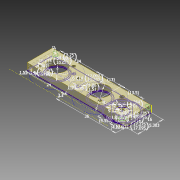
# Autodesk Inventor part: mount
Saved by Autodesk Inventor 2014 (Build 180170000, 170)
## iProperties
Created: 2013-09-13
Part Number: mount
Material: Nylon 6/6
Document SubType Name: Modeling
Designer: Brandon
Density: 1 g/cm^3
Appearance: Nylon 6
Author: Brandon
Autodesk Inventor part; units mm, degrees
ref_plane "YZ Plane" through (0, 0, 0) normal (1, 0, 0) x (0, 1, 0)
ref_plane "XZ Plane" through (0, 0, 0) normal (0, 1, 0) x (-1, 0, 0)
ref_plane "XY Plane" through (0, 0, 0) normal (0, 0, 1) x (1, 0, 0)
sketch "Sketch1" plane through (0, 0, 0) normal (0, 0, 1) x (1, 0, 0)
  circle A0 centre (0, 0) radius 0.88
  circle A1 centre (-13, 0) radius 6.031
  line L0 (0, 8.1062) -> (0, -7.1967)
  line L1 (-24, -7.1967) -> (0, -7.1967)
  line L2 (-24, 8.1062) -> (-24, -7.1967)
  circle A2 centre (-13, 0) radius 5.1925
  line L3 (-13, 0) -> (-9.1435, 0) construction
  line L4 (-13, 0) -> (-13, 0) construction
  circle A3 centre (-7.9046, 5.0954) radius 0.8375
  circle A4 centre (-18.0954, -5.0954) radius 0.8375
  circle A5 centre (13, 0) radius 6.031
  circle A6 centre (13, 0) radius 5.1925
  line L5 (13, 0) -> (9.1435, 0) construction
  line L6 (13, 0) -> (13, 0) construction
  circle A7 centre (7.9046, 5.0954) radius 0.8375
  circle A8 centre (18.0954, -5.0954) radius 0.8375
  line L7 (13, 0) -> (-13, 0)
  circle A9 centre (26.5, 0) radius 4.5 construction
  circle A10 centre (26.5, 0) radius 8.6375
  line L8 (26.5, 0) -> (30.5894, 0) construction
  circle A11 centre (22.8938, 3.6062) radius 1.132
  circle A12 centre (30.1062, -3.6062) radius 1.132
  line L9 (0, -7.1967) -> (-0.0026, -8.7967) construction
  line L10 (-0.0026, -8.7967) -> (-19.5634, -8.7649) construction
  line L11 (-0.0026, -8.7967) -> (19.5499, -8.8284) construction
  circle A13 centre (13, 0) radius 9 construction
  circle A14 centre (26.5, 0) radius 3.2675
  line L12 (13, 0) -> (26.5, 0)
  line L13 (30.1062, -3.6062) -> (22.8938, 3.6062) construction
  line L14 (33.2882, -0.4243) -> (26.0757, 6.7882)
  line L15 (19.7118, 0.4243) -> (26.9243, -6.7882)
  arc A15 (26.9243, -6.7882) -> (33.2882, -0.4243) centre (30.1062, -3.6062) ccw
  arc A16 (26.0757, 6.7882) -> (19.7118, 0.4243) centre (22.8938, 3.6062) ccw
  circle A17 centre (26.5, 0) radius 8
  circle A18 centre (26.5, 0) radius 3.5
  line L16 (-24, 8.1062) -> (0, 8.1062)
  line L17 (36, 8.1062) -> (36, -7.1967)
  line L18 (21.7235, -7.1967) -> (31.2765, -7.1967) construction
  line L19 (-0.0026, -8.7967) -> (-0.0018, -11.9967) construction
  line L20 (-0.0018, -11.9967) -> (30.0022, -11.9889) construction
  line L21 (-0.0018, -11.9967) -> (-29.9998, -12.0044) construction
  line L22 (-0.0018, -11.9967) -> (29.9963, -11.9967) construction
  circle A19 centre (0, 0) radius 4 construction
  line L23 (-13, 0) -> (-8.7354, 4.2646) construction
  line L24 (-13, 0) -> (-17.2646, -4.2646) construction
  line L25 (-8.7354, 4.2646) -> (-7.9046, 5.0954) construction
  line L26 (-17.2646, -4.2646) -> (-18.0954, -5.0954) construction
  line L27 (-17.2646, -4.2646) -> (-16.0896, -4.2646) construction
  circle A20 centre (13, 0) radius 12 construction
  circle A21 centre (-13, 0) radius 12 construction
  line L28 (1, 0) -> (-1, 0) construction
  line L29 (-19.031, 0) -> (-24, 0) construction
  line L30 (0, 8.1062) -> (36, 8.1062)
  line L31 (0, -7.1967) -> (36, -7.1967)
  line L32 (36, -7.1967) -> (36, -11.3938) construction
  circle A22 centre (22.8938, 3.6062) radius 1.9
  circle A23 centre (30.1062, -3.6062) radius 1.9
  dimension "d105" = 24
  dimension "d106" = 24
  dimension "d0" = 1.5
  dimension "d3" = 11.6
  dimension "d8" = 10
  dimension "d14" = 1.55
  dimension "d26" = 17
  dimension "d31" = 2
  dimension "d32" = 2
  dimension "d40" = 6.15
  dimension "d42" = 13
  dimension "d52" = 13.5
  dimension "d53" = 9
  dimension "d54" = 7
  dimension "d81" = 1.6
  dimension "d86" = 3.2
  dimension "d87" = 45
  dimension "d88" = 10.2
  dimension "d89" = 8
  dimension "d91" = 1.175
  dimension "d92" = 135
  dimension "d103" = 18
  dimension "d104" = 9
  dimension "d107" = 2
  dimension "d108" = 4.969
  dimension "d117" = 24
  dimension "d118" = 24
  dimension "d119" = 36
  dimension "d131" = 16
  dimension "d132" = 9.5529
  dimension "d133" = 4.7236
  dimension "d134" = 15.3029
  dimension "d135" = 3.8
  dimension "d136" = 3.8
  constraints: 68 end point, 22 centre point, 15 coincident, 10 horizontal, 9 point on circle, 7 collinear, 7 point on line, 7 tangent, 6 perpendicular, 6 symmetric about line, 3 equal length, 2 horizontal alignment, 2 midpoint, 1 equal radius, 1 parallel, 9 other
  measures "d42" distance of point (0, 0) A5.centre
  measures "d52" distance of L12.start L8.start
  measures "d53" diameter of A16
  measures "d54" diameter of A18
  measures "d81" distance of L9.end L0.end
  measures "d86" distance of L9.end L19.end
  measures "d87" angle of L8 L13
  measures "d88" distance of L13.start L13.end
  measures "d89" diameter of A19
  measures "d91" distance of L24.end L26.end
  measures "d92" angle of L26 L27
  measures "d103" diameter of A13
  measures "d104" diameter of A9
  measures "d107" distance of L28.start L28.end
  measures "d108" distance of L29.start L29.end
  measures "d117" distance of L2.start L0.start
  measures "d118" distance of L1.start L0.end
  measures "d119" distance of L0.end L17.end
  measures "d131" diameter of A17
  measures "d132" distance of L18.end L18.start
  measures "d133" distance of L17.end L18.end
  measures "d134" distance of L17.start L17.end
  measures "d135" diameter of A22
  measures "d136" diameter of A23
extrude "Extrusion5" add sketch "Sketch1" along normal blind 4 contours L7 L0 A0 | L7 A5 A10 L31 L0 A0 | A0 L0 L30 A16 A10 A5 L7 | A0 L0 L7 | L0 L7 A0 | A0 L0 L1 L2 L16 | A0 L7 L0 | L7 A6 A10 A5 | A5 A10 A6 L7 | A10 A16 A5 | A5 A17 L12 A6 A10 | A10 A6 L12 A17 A5 | A5 A17 L31 A10 | L30 A10 A16 | A16 A10 | A16 A17 A5 | A16 A10 A17 | A17 L12 A5 | A5 L12 L15 A15 L31 A17 | A10 L30 A15 A17 A16 | A17 A16 L15 L12 A5 | A5 L12 A17 | A17 A16 L14 A15 L31 L15 | A17 A15 L14 A16 | L30 L17 L31 A15 A10 | L31 A17 A15 A10 | A10 A15 L31 | A1 | A18 A22 | A23 A18 picked at (33.3877, -4.4134) picked at (32.25, -6.8178)
extrude "Extrusion6" add sketch "Sketch1" along normal blind 0.6 contours A14 A22 A18 A23 | A14 A22 A18 | A23 A18 A14 | A14 L12 A18 A22 | A23 A18 L12 A14
extrude "Extrusion7" add sketch "Sketch1" against normal blind 1 contours A17 L12 A5 | A5 L12 L15 A15 L31 A17 | L31 A15 A17 | A17 A16 L15 L12 A5 | A5 L12 A17 | A17 A16 L14 A15 L31 L15 | A17 A15 L14 A16 | A15 L31 A17 | A14 A22 A18 A23 | A14 A22 A18 | A23 A18 A14 | A14 L12 A18 A22 | A18 A22 | A23 A18 L12 A14 | A23 A18
extrude "Extrusion8" add sketch "Sketch1" against normal blind 2 contours A16 A10 | A16 A10 A17 | A15 A17 L31 A10 | A10 L31 A15 | A17 A16 L14 A15 L31 L15 | L31 A17 A15 A10 | A10 A15 L31 | A15 L31 A17 | A14 A22 A18 A23 | A14 A22 A18 | A23 A18 A14 | A14 L12 A18 A22 | A18 A22 | A23 A18 L12 A14 | A23 A18 picked at (30.6666, -7.3082) picked at (33.3877, -4.4134) picked at (28.3667, -7.2701)
extrude "Extrusion9" cut sketch "Sketch1" against normal up to surface (1 mm away) from surface at -1 contours A10 A16 A5 | A5 A17 L12 A6 A10 | A10 A6 L12 A17 A5 | A5 A17 L31 A10 | A16 A17 A5 | A16 A10 A17 | A6 L12 A10 | A17 L12 A5 | A5 L12 L15 A15 L31 A17 | A10 L12 A6 | A10 L30 A15 A17 A16 | A10 L30 | A17 A16 L15 L12 A5 | A5 L12 A17 | A17 A16 L14 A15 L31 L15 | A17 A15 L14 A16 | L31 A17 A15 A10 | A14 A22 A18 A23 | A14 A22 A18 | A23 A18 A14 | A14 L12 A18 A22 | A18 A22 | A23 A18 L12 A14 | A23 A18 picked at (33.3877, -4.4134)
extrude "Extrusion10" cut sketch "Sketch1" against normal blind 2 contours L7 L0 A0 | L7 A5 A10 L31 L0 A0 | A0 L0 L30 A16 A10 A5 L7 | A0 L0 L7 | A10 A16 A5 | A5 A17 L31 A10 | L30 A10 A16 | A16 A10 | A16 A17 A5 | A16 A10 A17 | A5 L12 L15 A15 L31 A17 | A10 L30 A15 A17 A16 | A17 A16 L15 L12 A5 | A17 A16 L14 A15 L31 L15 | A17 A15 L14 A16 | L30 L17 L31 A15 A10 | L31 A17 A15 A10 | A10 A15 L31 | A18 A22 | A23 A18 keep common part picked at (0.4122, 0.4122) picked at (0.4122, -0.4122) picked at (33.3877, -4.4134) picked at (32.25, -6.8178)
extrude "Extrusion11" add sketch "Sketch1" along normal blind 4 contours L7 L0 A0 | L7 A5 A10 L31 L0 A0 | A0 L0 L30 A16 A10 A5 L7 | A0 L0 L7 | L0 L7 A0 | A0 L0 L1 L2 L16 | A0 L7 L0 | L7 A6 A10 A5 | A5 A10 A6 L7 | A10 A16 A5 | A5 A17 L12 A6 A10 | A10 A6 L12 A17 A5 | A5 A17 L31 A10 | L30 A10 A16 | A16 A10 | A16 A17 A5 | A16 A10 A17 | A17 L12 A5 | A5 L12 L15 A15 L31 A17 | A10 L30 A15 A17 A16 | A17 A16 L15 L12 A5 | A5 L12 A17 | A17 A16 L14 A15 L31 L15 | A17 A15 L14 A16 | L30 L17 L31 A15 A10 | L31 A17 A15 A10 | A10 A15 L31 | A1 | A18 A22 | A23 A18 picked at (33.3877, -4.4134) picked at (32.25, -6.8178)
extrude "Extrusion12" add sketch "Sketch1" against normal blind 1 contours A14 A22 A18 A23 | A14 A22 A18 | A23 A18 A14 | A14 L12 A18 A22 | A23 A18 L12 A14
extrude "Extrusion13" add sketch "Sketch1" along normal blind 0.5 contours A14 A22 A18 A23 | A14 A22 A18 | A23 A18 A14 | A14 L12 A18 A22 | A23 A18 L12 A14
extrude "Extrusion14" cut sketch "Sketch1" along normal blind 0.9 contours L7 A6 A10 A5 | A5 A10 A6 L7 | A5 A17 L12 A6 A10 | A10 A6 L12 A17 A5 | A17 L12 A5 | A5 L12 A17 | A1
extrude "Extrusion15" cut sketch "Sketch1" along normal blind 10 contours L7 L0 A0 | A0 L0 L7 | L0 L7 A0 | A0 L7 L0
sketch "Sketch2" plane through (-24, 8.1062, 0) normal (0, 1, 0) x (1, 0, 0)
  line L0 (1.4823, 0) -> (0, 0)
  circle A0 centre (2, -2) radius 1.375
  circle A1 centre (58, -2) radius 1.375
  line L1 (0, 0) -> (0, -4) projected
  line L2 (60, 0) -> (60, -4) projected
  line L3 (2, -2) -> (0, -2) construction
  line L4 (58, -2) -> (60, -2) construction
  dimension "d126" = 2.5
  dimension "d128" = 2
  constraints: 6 end point, 2 centre point, 2 midpoint, 1 collinear, 1 equal radius
  measures "d128" distance of L3.start L3.end
extrude "Extrusion16" cut sketch "Sketch2" against normal up to next contours A0
extrude "Extrusion17" cut sketch "Sketch2" against normal up to next contours A1
chamfer "Chamfer1" distance 1 angle 45 2 edges at (28.9742, -3.6062, 4) (21.7618, 3.6062, 4)
body "Solid3"
